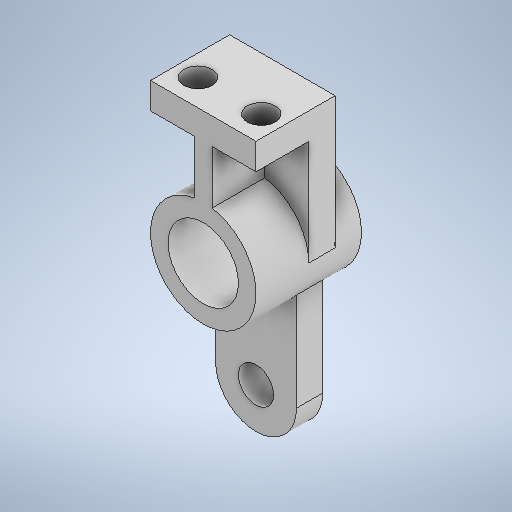
# Autodesk Inventor part: cad@71
Saved by Autodesk Inventor 2025.2 (Build 292293000, 293)
## iProperties
Created: 2025-04-22
Part Number: cad@71
Material: Generic
Document SubType Name: Modeling
Designer: spars
Density: 1 g/cm^3
Appearance: Default
Author: spars
Autodesk Inventor part; units mm, degrees
ref_plane "YZ Plane" through (0, 0, 0) normal (1, 0, 0) x (0, 1, 0)
ref_plane "XZ Plane" through (0, 0, 0) normal (0, 1, 0) x (-1, 0, 0)
ref_plane "XY Plane" through (0, 0, 0) normal (0, 0, 1) x (1, 0, 0)
sketch "Sketch1" plane through (0, 0, 0) normal (0, 0, 1) x (1, 0, 0)
  line L0 (-30, 37.5) -> (30, 37.5)
  line L1 (30, 37.5) -> (30, -37.5)
  line L2 (30, -37.5) -> (-30, -37.5)
  line L3 (-30, -37.5) -> (-30, 37.5)
  line L4 (-30, 37.5) -> (30, -37.5) construction
  line L5 (30, 37.5) -> (-30, -37.5) construction
  circle A0 centre (0, -37.5) radius 30
  circle A1 centre (0, -37.5) radius 20
  circle A2 centre (0, -112.5) radius 23
  circle A3 centre (0, -112.5) radius 10
  line L6 (-23, -112.5) -> (-23, -56.7614)
  line L7 (23, -112.5) -> (23, -56.7614)
  line L8 (-30, 37.5) -> (30, 37.5)
  line L9 (30, 37.5) -> (30, 22.5)
  line L10 (30, 22.5) -> (-30, 22.5)
  line L11 (-30, 22.5) -> (-30, 37.5)
  line L12 (-5, 22.5) -> (5, 22.5)
  line L13 (5, 22.5) -> (5, -7.9196)
  line L14 (-5, -7.9196) -> (-5, 22.5)
  point P0 (0, 0)
  dimension "d0" = 60
  dimension "d1" = 75
  dimension "d2" = 60
  dimension "d3" = 40
  dimension "d4" = 46
  dimension "d5" = 20
  dimension "d6" = 75
  dimension "d7" = 15
  dimension "d9" = 25
  constraints: 30 end point, 6 parallel, 6 point on circle, 4 centre point, 3 horizontal, 3 midpoint, 3 perpendicular, 2 coincident, 2 point on line, 2 tangent, 1 vertical
  measures "d0" distance of L1.end L2.end
  measures "d1" distance of L0.end L1.end
  measures "d2" diameter of A0
  measures "d3" diameter of A1
  measures "d4" diameter of A2
  measures "d5" diameter of A3
  measures "d6" distance of A2.centre A0.centre
  measures "d7" distance of L8.end L9.end
  measures "d9" distance between parallel lines of L3 L14
extrude "Extrusion1" add sketch "Sketch1" along normal blind 15 contours L10 L14 A0 L3 | L1 A0 L13 L10 | A0 L7 A2 L6 | A2
extrude "Extrusion2" add sketch "Sketch1" along normal blind 45 contours L0 L1 L10 L3 | L10 L13 A0 L14
extrude "Extrusion3" add sketch "Sketch1" along normal blind 45 and the other way blind 15 contours A0 L2 A1 | L2 A1 A0
sketch "Sketch2" plane through (-30, 22.5, 15) normal (0, -1, 0) x (1, 0, 0)
  point P0 (30, -15)
sketch "Sketch3" plane through (-30, 22.5, 15) normal (0, -1, 0) x (1, 0, 0)
  point P0 (30, -15)
sketch "Sketch4" plane through (-30, 37.5, 0) normal (0, 1, 0) x (1, 0, 0)
  circle A0 centre (12, -30) radius 8
  line L0 (0, 0) -> (0, -45) projected
  line L1 (60, -45) -> (0, -45) projected
  circle A1 centre (48, -30) radius 8
  point P0 (30, 0)
  dimension "d18" = 16
  dimension "d19" = 12
  dimension "d20" = 15
  constraints: 2 centre point
  measures "d18" diameter of A0
  measures "d19" distance from line of L0 A0.centre
  measures "d20" distance from line of L1 A0.centre
extrude "Extrusion4" cut sketch "Sketch4" against normal blind 15
body "Solid1"
